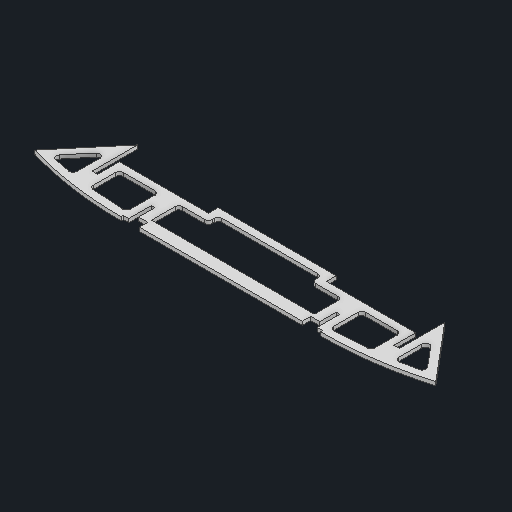
# Autodesk Inventor part: tail_1
Saved by Autodesk Inventor 2023 (Build 270158030, 158C)
## iProperties
Created: 2022-03-21
Part Number: tail_1
Material: Generic
Document SubType Name: Modeling
Designer: kardo
Density: 1 g/cm^3
Appearance: Default
Mass: 2.78715 g
Surface Area: 39.0166 cm^2
Volume: 2.78715 cm^3
Author: kardo
Autodesk Inventor part; units mm, degrees
ref_plane "YZ Plane" through (0, 0, 0) normal (1, 0, 0) x (0, 1, 0)
ref_plane "XZ Plane" through (0, 0, 0) normal (0, 1, 0) x (-1, 0, 0)
ref_plane "XY Plane" through (0, 0, 0) normal (0, 0, 1) x (1, 0, 0)
derived "parameters_frame.ipt"
derived "stencil_frame.ipt"
sketch "sk_joint_locations" plane through (81.12, 0, 0) normal (1, 0, 0) x (0, 1, 0)
  line L0 (0, 0) -> (111.39, 7.7891) construction
  line L1 (30.81, 28.832) -> (94.8, 28.832) construction
  arc A0 (30.81, 28.832) -> (9.48, 28.5282) centre (30.81, -720.1791) ccw construction
  line L2 (-254.1001, 21.0191) -> (9.48, 28.5282) construction
  line L3 (-363, 18.496) -> (-275.8801, 20.463) construction
  arc A1 (-275.8801, 20.463) -> (-254.1001, 21.0191) centre (-359.1231, 3707.4463) ccw construction
  line L4 (-210.8824, 4616.4994) -> (225.0382, -1617.4555) construction
  line L5 (-242.0001, 4592.9714) -> (-242.0001, -1605.7041) construction
  line L6 (-120.9999, 4592.9714) -> (-120.9999, -1605.7041) construction
  line L7 (-363, 4592.9714) -> (-363, -1605.7041) construction
  line L8 (0, 4592.9714) -> (0, -1605.7041) construction
  line L9 (551.8244, 47.4419) -> (-603.6686, 7.0912) construction
  line L10 (-657.8036, -26.1228) -> (709.4042, 69.4817) construction
  line L11 (178.2183, 30.3929) -> (177.9391, 38.388) construction
  line L12 (185.9231, 36.8959) -> (186.4825, 28.8959) construction
  line L13 (0, 6.528) -> (111.1168, 11.6964) construction
  line L14 (-242.0001, 45.8501) -> (-242.0001, 21.3638) construction
  line L15 (-363, 37.4293) -> (-363, 18.496) construction
  line L16 (-120.9999, 51.0063) -> (-120.9999, 24.811) construction
  line L17 (0, 52.89) -> (0, 28.2581) construction
  line L18 (108.3896, 50.6971) -> (108.935, 42.897) construction
  line L19 (109.4805, 35.0968) -> (108.935, 42.897) construction
  line L20 (109.4805, 35.0968) -> (110.0259, 27.2967) construction
  line L21 (110.0259, 27.2967) -> (110.5713, 19.4965) construction
  line L22 (110.5713, 19.4965) -> (111.1168, 11.6964) construction
  line L23 (0, 6.528) -> (0, 0) construction
  spline S0 degree 4 poles (-363, 37.4293) (-272.3626, 45.1427) (-181.5879, 49.7528) (-90.8131, 52.89) (0, 52.89) knots 0 0 0 0 0 1 1 1 1 1
  spline S1 degree 3 poles (0, 52.89) (86.3106, 52.89) (181.3207, 49.5034) (237, 36.448) knots 0 0 0 0 1 1 1 1
  spline S2 degree 2 poles (111.39, 7.7891) (176.0348, 12.3096) (237, 36.448) knots 0 0 0 1 1 1
  line L24 (94.8, 37.536) -> (94.8, 28.832) construction
  line L25 (94.8, 35.548) -> (94.8, 30.82) construction
  point P0 (-210.8824, 4616.4994)
  point P1 (225.0382, -1617.4555)
  point P2 (178.0787, 34.3904)
  point P3 (186.2028, 32.8959)
  point P4 (134.9575, 11.3411)
  point P5 (-363, 27.9627)
  point P6 (-242.0001, 33.6069)
  point P7 (-120.9999, 37.9086)
  point P8 (0, 40.5741)
  point P9 (94.8, 33.184)
sketch "sk_cowl_joint_locations" plane through (54.6, 0, 0) normal (1, 0, 0) x (0, 1, 0)
  line L0 (-363, 18.496) -> (-275.8801, 20.463) construction
  arc A0 (-275.8801, 20.463) -> (-254.1001, 21.0191) centre (-359.1231, 3707.4463) ccw construction
  line L1 (-254.1001, 21.0191) -> (9.48, 28.5282) construction
  arc A1 (30.81, 28.832) -> (9.48, 28.5282) centre (30.81, -720.1791) ccw construction
  line L2 (30.81, 28.832) -> (94.8, 28.832) construction
  line L3 (94.8, 30.032) -> (30.81, 30.032) construction
  arc A2 (30.81, 30.032) -> (9.4458, 29.7277) centre (30.81, -720.1791) ccw construction
  line L4 (9.4458, 29.7277) -> (-254.1343, 22.2186) construction
  arc A3 (-275.9072, 21.6626) -> (-254.1343, 22.2186) centre (-359.1231, 3707.4463) ccw construction
  line L5 (-275.9072, 21.6626) -> (-363, 19.6963) construction
  line L6 (-242.0001, 4592.9714) -> (-242.0001, -1605.7041) construction
  line L7 (-120.9999, 4592.9714) -> (-120.9999, -1605.7041) construction
  line L8 (-363, 4592.9714) -> (-363, -1605.7041) construction
  line L9 (0, 4592.9714) -> (0, -1605.7041) construction
  line L10 (-242.0001, 45.0688) -> (-242.0001, 22.5643) construction
  line L11 (-120.9999, 49.9661) -> (-120.9999, 26.0115) construction
  line L12 (-363, 19.6963) -> (-363, 19.6963)
  line L13 (-363, 19.6963) -> (-363, 36.9211) construction
  line L14 (-1229.7832, 4422.8213) -> (280.3081, -1633.8241) construction
  line L15 (-362.7741, 36.9211) -> (-363, 39.712) construction
  line L16 (0, 51.6) -> (0, 29.4586) construction
  spline S0 degree 2 poles (-363, 39.712) (-181.6483, 54.394) (0, 54.4) knots 0 0 0 1 1 1
  spline S1 degree 3 poles (0, 54.4) (31.284, 54.4) (68.256, 47.9917) (94.8, 37.536) knots 1 1 1 1 2 2 2 2
  spline S2 degree 3 poles (93.7738, 34.9308) (89.4268, 36.6431) (81.2968, 39.4556) (71.234, 42.2519) (63.4432, 44.1558) (58.1419, 45.3261) (51.4169, 46.6598) (45.9725, 47.6212) (39.1225, 48.6857) (33.6211, 49.4253) (26.7536, 50.2046) (21.2812, 50.7098) (14.5037, 51.1886) (7.8073, 51.5121) (2.5751, 51.6) (0, 51.6) knots 1 1 1 1 1.166667 1.291667 1.333333 1.416667 1.458333 1.541667 1.583333 1.666667 1.708333 1.791667 1.833333 1.916667 2 2 2 2
  spline S3 degree 3 poles (0, 51.6) (-20.1706, 51.5993) (-55.4643, 51.3605) (-95.7903, 50.6123) (-126.0307, 49.8474) (-146.1889, 49.2356) (-171.3841, 48.3435) (-191.5382, 47.528) (-216.7283, 46.3813) (-236.8783, 45.3621) (-262.0632, 43.9608) (-282.2091, 42.7379) (-307.3889, 41.082) (-332.5661, 39.2987) (-352.7052, 37.7363) (-362.7741, 36.9211) knots 0 0 0 0 0.166667 0.291667 0.333333 0.416667 0.458333 0.541667 0.583333 0.666666 0.708333 0.791666 0.833333 0.916666 1 1 1 1
  line L17 (-142.5135, 45.4866) -> (-137.5404, 25.5402) construction
  line L18 (-134.9025, 31.4945) -> (-138.7836, 30.5268) construction
  line L19 (-137.3891, 41.4677) -> (-141.2702, 40.5) construction
  line L20 (-142.5135, 45.4866) -> (-138.6324, 46.4543) construction
  line L21 (-137.5404, 25.5402) -> (-133.6592, 26.5079) construction
  line L22 (-138.6324, 46.4543) -> (-138.8117, 52.2515) construction
  point P0 (0, 0)
  point P1 (-363, 28.3087)
  point P2 (-242.0001, 33.8165)
  point P3 (-120.9999, 37.9888)
  point P4 (0, 40.5293)
  point P5 (-1229.7832, 4422.8213)
  point P6 (280.3081, -1633.8241)
  point P7 (-85.2629, 50.788)
  point P8 (0, 40.5293)
sketch "sk_tail_1_base" plane through (0, -120.9999, 0) normal (0, 1, 0) x (-1, 0, 0)
  spline S0 degree 2 poles (-156, 24.8232) (-108.135, 52.7671) (-54.6, 52.7671) knots 0 0 0 1 1 1 construction
  line L0 (-54.6, 52.7671) -> (0, 52.7671) construction
  line L1 (0, -1605.7041) -> (0, 4592.9714) construction
  line L2 (759.9345, -994.7137) -> (-2384.2453, 2752.3738) construction
  line L3 (-109.794, 43.6552) -> (-84.12, 13.0581)
  line L4 (-84.12, 13.0581) -> (-84.12, 37.9086)
  line L5 (-84.12, 37.9086) -> (-81.12, 37.9086)
  line L6 (-81.12, 37.9086) -> (-81.12, 26.011)
  line L7 (-81.12, 26.011) -> (-32.32, 26.011)
  line L8 (-32.32, 26.011) -> (-32.32, 20.7064)
  line L9 (-32.32, 20.7064) -> (0, 20.7064)
  line L10 (0, 20.7064) -> (0, 51.5671)
  line L11 (-54.6, 51.5671) -> (0, 51.5671)
  spline S1 degree 5 poles (-155.395, 23.7869) (-146.1727, 29.1709) (-136.6335, 34.0111) (-126.7928, 38.2391) (-106.7786, 45.2706) (-85.9951, 49.5098) (-75.5682, 50.8937) (-65.0842, 51.567) (-54.6, 51.5671) knots 0 0 0 0 0 0 0.504597 0.504597 0.504597 1 1 1 1 1 1
  point P0 (0, 0)
  point P1 (-34.32, 24.811)
  point P2 (-34.32, 19.5064)
  dimension "d8" = 1.2
  dimension "d3" = 1.2
  dimension "d4" = 1.2
  dimension "d5" = 2
  dimension "d6" = 3
  dimension "d7" = 1.2
  constraints: 18 end point, 5 parallel, 3 perpendicular, 2 point on line, 4 other
  measures "d3" distance from line of point (-34.32, 19.506) L9
  measures "d4" distance from line of L7 point (-34.32, 24.811)
  measures "d5" distance from line of point (-34.32, 24.811) L8
  measures "d6" distance of L4.end L5.end
  measures "d7" distance between parallel lines of L2 L3
extrude "thicken" add sketch "sk_tail_1_base" along normal blind 2
sketch "sk_cut_stringer_cowl" plane through (0, -120.9999, 0) normal (0, 1, 0) x (-1, 0, 0)
  line L0 (-54.6, -1605.7041) -> (-54.6, 4592.9714) construction
  line L1 (-54.6, 52.7671) -> (0, 52.7671) projected
  line L2 (-49.6, 52.7671) -> (-49.6, 37.9888)
  line L3 (-49.6, 37.9888) -> (-51.6, 37.9888)
  line L4 (-51.6, 37.9888) -> (-51.6, 52.7671)
  point P0 (0, 0)
  point P1 (-54.6, 37.9888)
  dimension "d11" = 2
  dimension "d12" = 5
  constraints: 6 end point, 3 point on line, 2 parallel
  measures "d11" distance between parallel lines of L4 L2
  measures "d12" distance between parallel lines of L0 L2
extrude "cut_joint" cut sketch "sk_cut_stringer_cowl" along normal through all both and the other way through all
sketch "sk_cut_cowl_liner" plane through (0, -120.9999, 0) normal (0, 1, 0) x (-1, 0, 0)
  line L0 (-54.6, 52.7671) -> (0, 52.7671) projected
  line L1 (-54.6, -1605.7041) -> (-54.6, 4592.9714) projected
  line L2 (-44.6, 52.7671) -> (-44.6, 46.9671)
  line L3 (-44.6, 46.9671) -> (-49.6, 46.9671)
  line L4 (-49.6, 46.9671) -> (-49.6, 50.3671)
  line L5 (-49.6, 50.3671) -> (-54.6, 50.3671)
  point P0 (0, 0)
  dimension "d15" = 5
  dimension "d16" = 5
  dimension "d17" = 2.4
  dimension "d38" = 5.8
  constraints: 8 end point, 4 parallel, 2 point on line
  measures "d15" distance between parallel lines of L4 L2
  measures "d16" distance of L4.end L5.end
  measures "d17" distance between parallel lines of L0 L5
  measures "d38" distance of L2.start L2.end
extrude "cut_liner" cut sketch "sk_cut_cowl_liner" along normal through all both and the other way through all
sketch "sk_cut_weight" plane through (0, -120.9999, 0) normal (0, 1, 0) x (-1, 0, 0)
  line L0 (-32.32, 20.7064) -> (0, 20.7064) construction
  line L1 (-32.32, 26.011) -> (-32.32, 20.7064) construction
  line L2 (-81.12, 26.011) -> (-32.32, 26.011) construction
  line L3 (-81.12, 37.9086) -> (-81.12, 26.011) construction
  line L4 (-49.6, 46.9671) -> (-49.6, 50.3671) construction
  line L5 (-44.6, 46.9671) -> (-49.6, 46.9671) construction
  line L6 (-44.6, 52.7671) -> (-44.6, 46.9671) construction
  spline S0 degree 3 poles (-155.395, 23.7869) (-152.7498, 25.3312) (-147.434, 28.2907) (-140.7253, 31.6676) (-133.9686, 34.803) (-128.5248, 37.118) (-121.6718, 39.7704) (-116.1508, 41.6992) (-109.2012, 43.8689) (-103.6026, 45.4118) (-96.5557, 47.0992) (-90.8792, 48.2563) (-82.3056, 49.7027) (-70.7692, 51.117) (-60.5135, 51.5671) (-54.6, 51.5671) knots 0 0 0 0 0.083333 0.166667 0.208333 0.291667 0.333333 0.416667 0.458333 0.541667 0.583333 0.666667 0.708333 0.833333 1 1 1 1 construction
  line L7 (0, -1605.7041) -> (0, 4592.9714) projected
  line L8 (0, 24.7064) -> (-28.32, 24.7064)
  line L9 (-28.32, 24.7064) -> (-28.32, 30.011)
  line L10 (-28.32, 30.011) -> (-44.6, 30.011)
  line L11 (-77.12, 30.011) -> (-77.12, 46.2948)
  line L12 (-77.12, 46.2948) -> (-55.6, 47.5671)
  line L13 (-55.6, 47.5671) -> (-55.6, 30.011)
  line L14 (-55.6, 30.011) -> (-77.12, 30.011)
  line L15 (-44.6, 44.9671) -> (-44.6, 30.011)
  line L16 (-44.6, 44.9671) -> (0, 44.9671)
  line L17 (-77.12, 46.2948) -> (-77.12, 50.2948) construction
  line L18 (-49.6, 46.9671) -> (-49.6, 26.011) construction
  line L19 (-49.6, 46.9671) -> (-51.6, 46.9671) construction
  line L20 (-51.6, 46.9671) -> (-51.6, 26.011) construction
  line L21 (-109.794, 43.6552) -> (-84.12, 13.0581) construction
  line L22 (-84.12, 13.0581) -> (-84.12, 37.9086) construction
  line L23 (-88.12, 24.048) -> (-88.12, 44.7158)
  line L24 (-88.12, 44.7158) -> (-103.0033, 41.7853)
  line L25 (-103.0033, 41.7853) -> (-88.12, 24.048)
  line L26 (-88.12, 44.7158) -> (-88.12, 48.7158) construction
  line L27 (-103.0033, 41.7853) -> (-105.5745, 44.8494) construction
  point P0 (0, 0)
  dimension "d21" = 4
  dimension "d22" = 2
  dimension "d23" = 4
  dimension "d24" = 4
  dimension "d25" = 4
  dimension "d27" = 2
  dimension "d28" = 4
  dimension "d29" = 4
  dimension "d30" = 4
  dimension "d31" = 4
  dimension "d35" = 4
  dimension "d36" = 4
  dimension "d37" = 4
  constraints: 36 end point, 12 parallel, 5 collinear, 4 point on line, 1 equal length, 1 perpendicular, 3 other
  measures "d21" distance of L11.end L17.end
  measures "d22" distance between parallel lines of L20 L18
  measures "d23" distance between parallel lines of L0 L8
  measures "d24" distance between parallel lines of L1 L9
  measures "d25" distance between parallel lines of L10 L2
  measures "d27" distance between parallel lines of L16 L5
  measures "d28" distance between parallel lines of L20 L13
  measures "d29" distance between parallel lines of L2 L14
  measures "d30" distance between parallel lines of L11 L3
  measures "d31" vertical distance of point (-54.6, 51.567) L12.end
  measures "d35" distance between parallel lines of L21 L25
  measures "d36" distance between parallel lines of L23 L22
  measures "d37" distance of L23.end L26.end
extrude "cut_weight" cut sketch "sk_cut_weight" along normal through all both and the other way through all
fillet "round_corners" radius 2 10 edges at (28.32, -119.9999, 24.7064) (28.32, -119.9999, 30.011) (77.12, -119.9999, 30.011) (55.6, -119.9999, 30.011) (44.6, -119.9999, 30.011) (77.12, -119.9999, 46.2948) (55.6, -119.9999, 47.5671) (103.0033, -119.9999, 41.7853) (88.12, -119.9999, 24.048) (88.12, -119.9999, 44.7158)
mirror "mirror" about plane through (0, 0, 0) normal (1, 0, 0)
equation "\"d8\" = shell_thickness"
equation "\"d3\" = shell_thickness"
equation "\"d4\" = shell_thickness"
equation "\"d5\" = bulkhead_thickness"
equation "\"d6\" = stringer_thickness"
equation "\"d7\" = shell_thickness"
equation "\"d9\" = bulkhead_thickness"
equation "\"d11\" = bulkhead_thickness"
equation "\"d12\" = cowl_liner_width"
equation "\"d15\" = cowl_sealing_width"
equation "\"d16\" = cowl_liner_width"
equation "\"d17\" = shell_thickness + cowl_liner_thickness"
equation "\"d38\" = cowl_sealing_thickness + cowl_shell_thickness + cowl_liner_thickness"
equation "\"d21\" = bulkhead_inset"
equation "\"d22\" = bulkhead_thickness"
equation "\"d23\" = bulkhead_inset"
equation "\"d24\" = bulkhead_inset"
equation "\"d25\" = bulkhead_inset"
equation "\"d28\" = bulkhead_inset"
equation "\"d29\" = bulkhead_inset"
equation "\"d30\" = bulkhead_inset"
equation "\"d31\" = bulkhead_inset"
equation "\"d35\" = bulkhead_inset"
equation "\"d36\" = bulkhead_inset"
equation "\"d37\" = bulkhead_inset"
equation "\"d34\" = 0.5 * bulkhead_inset"
equation "\"shell_thickness\" = 1.2"
equation "\"stringer_thickness\" = 3"
equation "\"bulkhead_thickness\" = 2"
equation "\"cowl_liner_width\" = 5"
equation "\"cowl_sealing_width\" = 5"
equation "\"cowl_liner_thickness\" = 1.2"
equation "\"cowl_sealing_thickness\" = 3"
equation "\"cowl_shell_thickness\" = 1.6"
equation "\"bulkhead_inset\" = 4"
body "Solid1"
